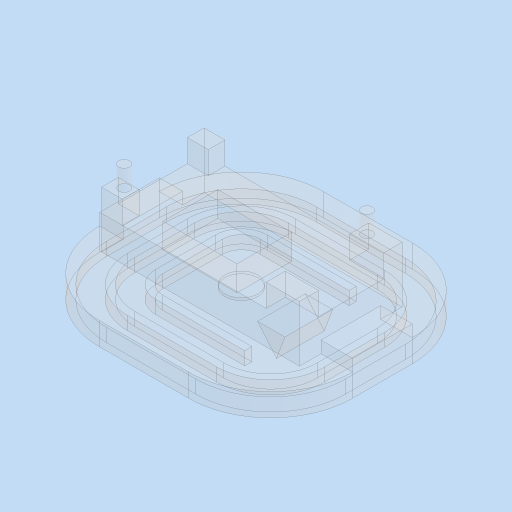
# Autodesk Inventor part: LM19-LSI_lens
Saved by Autodesk Inventor 2024 (Build 280153000, 153)
## iProperties
Created: 2025-05-08
Part Number: LM19-LSI_lens
Material: Polycarbonate, Clear
Document SubType Name: Modeling
Designer: XxPan
Density: 1.2 g/cm^3
Appearance: Polycarbonate - Clear
Author: XxPan
Autodesk Inventor part; units mm, degrees
ref_plane "YZ Plane" through (0, 0, 0) normal (1, 0, 0) x (0, 1, 0)
ref_plane "XZ Plane" through (0, 0, 0) normal (0, 1, 0) x (-1, 0, 0)
sketch "Sketch1" plane through (0, 0, 0) normal (0, 1, 0) x (-1, 0, 0)
  line L0 (3.725, 9.375) -> (-3.725, 9.375)
  line L1 (-10.6, 2.5) -> (-10.6, -2.5)
  line L2 (-3.725, -9.375) -> (3.725, -9.375)
  line L3 (10.6, -2.5) -> (10.6, 2.5)
  line L4 (16.8334, 0) -> (-16.8334, 0) construction
  line L5 (0, -15.1184) -> (0, 15.1184) construction
  arc A0 (10.6, 2.5) -> (3.725, 9.375) centre (3.725, 2.5) ccw
  arc A1 (3.725, -9.375) -> (10.6, -2.5) centre (3.725, -2.5) ccw
  arc A2 (-10.6, -2.5) -> (-3.725, -9.375) centre (-3.725, -2.5) ccw
  arc A3 (-3.725, 9.375) -> (-10.6, 2.5) centre (-3.725, 2.5) ccw
  point P0 (0, 0)
  point P1 (-10.6, -9.375)
  point P2 (-10.6, 9.375)
  point P3 (10.6, -9.375)
  dimension "d0" = 21.2
  dimension "d1" = 18.75
  dimension "d2" = 6.875
  constraints: 8 end point, 8 point on circle, 8 tangent, 6 point on line, 4 centre point, 3 equal radius, 2 parallel, 1 horizontal, 1 perpendicular, 2 other
  measures "d0" distance of point (10.6, -9.375) point (-10.6, -9.375)
  measures "d1" distance of point (-10.6, -9.375) point (-10.6, 9.375)
  measures "d2" radius of A0
extrude "Extrusion1" add sketch "Sketch1" against normal blind 0.8
sketch "Sketch2" plane through (0, -0.8, 0) normal (0, -1, 0) x (1, 0, 0)
  line L0 (10.6, -2.5) -> (10.6, 2.5) projected
  arc A0 (10.6, 2.5) -> (3.725, 9.375) centre (3.725, 2.5) ccw projected
  arc A1 (3.725, -9.375) -> (10.6, -2.5) centre (3.725, -2.5) ccw projected
  line L1 (-3.725, -9.375) -> (3.725, -9.375) projected
  arc A2 (-10.6, -2.5) -> (-3.725, -9.375) centre (-3.725, -2.5) ccw projected
  line L2 (-10.6, 2.5) -> (-10.6, -2.5) projected
  arc A3 (-3.725, 9.375) -> (-10.6, 2.5) centre (-3.725, 2.5) ccw projected
  line L3 (3.725, 9.375) -> (-3.725, 9.375) projected
  arc A4 (10, 2.5) -> (3.725, 8.775) centre (3.725, 2.5) ccw
  line L4 (10, 2.5) -> (10, -2.5)
  arc A5 (3.725, -8.775) -> (10, -2.5) centre (3.725, -2.5) ccw
  line L5 (3.725, -8.775) -> (-3.725, -8.775)
  arc A6 (-10, -2.5) -> (-3.725, -8.775) centre (-3.725, -2.5) ccw
  line L6 (-10, -2.5) -> (-10, 2.5)
  arc A7 (-3.725, 8.775) -> (-10, 2.5) centre (-3.725, 2.5) ccw
  line L7 (-3.725, 8.775) -> (3.725, 8.775)
  arc A8 (8.25, 2.5) -> (3.725, 7.025) centre (3.725, 2.5) ccw
  line L8 (8.25, 2.5) -> (8.25, -2.5)
  arc A9 (3.725, -7.025) -> (8.25, -2.5) centre (3.725, -2.5) ccw
  line L9 (3.725, -7.025) -> (-3.725, -7.025)
  arc A10 (-8.25, -2.5) -> (-3.725, -7.025) centre (-3.725, -2.5) ccw
  line L10 (-8.25, -2.5) -> (-8.25, 2.5)
  arc A11 (-3.725, 7.025) -> (-8.25, 2.5) centre (-3.725, 2.5) ccw
  line L11 (-3.725, 7.025) -> (3.725, 7.025)
  arc A12 (7.65, 2.5) -> (3.725, 6.425) centre (3.725, 2.5) ccw
  line L12 (7.65, 2.5) -> (7.65, -2.5)
  arc A13 (3.725, -6.425) -> (7.65, -2.5) centre (3.725, -2.5) ccw
  line L13 (3.725, -6.425) -> (-3.725, -6.425)
  arc A14 (-7.65, -2.5) -> (-3.725, -6.425) centre (-3.725, -2.5) ccw
  line L14 (-7.65, -2.5) -> (-7.65, 2.5)
  arc A15 (-3.725, 6.425) -> (-7.65, 2.5) centre (-3.725, 2.5) ccw
  line L15 (-3.725, 6.425) -> (3.725, 6.425)
  arc A16 (5.9, 2.5) -> (3.725, 4.675) centre (3.725, 2.5) ccw
  line L16 (5.9, 2.5) -> (5.9, -2.5)
  arc A17 (3.725, -4.675) -> (5.9, -2.5) centre (3.725, -2.5) ccw
  line L17 (3.725, -4.675) -> (-3.725, -4.675)
  arc A18 (-5.9, -2.5) -> (-3.725, -4.675) centre (-3.725, -2.5) ccw
  line L18 (-5.9, -2.5) -> (-5.9, 2.5)
  arc A19 (-3.725, 4.675) -> (-5.9, 2.5) centre (-3.725, 2.5) ccw
  line L19 (-3.725, 4.675) -> (3.725, 4.675)
  arc A20 (5.3, 2.5) -> (3.725, 4.075) centre (3.725, 2.5) ccw
  line L20 (5.3, 2.5) -> (5.3, -2.5)
  arc A21 (3.725, -4.075) -> (5.3, -2.5) centre (3.725, -2.5) ccw
  line L21 (3.725, -4.075) -> (-3.725, -4.075)
  arc A22 (-5.3, -2.5) -> (-3.725, -4.075) centre (-3.725, -2.5) ccw
  line L22 (-5.3, -2.5) -> (-5.3, 2.5)
  arc A23 (-3.725, 4.075) -> (-5.3, 2.5) centre (-3.725, 2.5) ccw
  line L23 (-3.725, 4.075) -> (3.725, 4.075)
  line L24 (3.725, 4.075) -> (3.725, 4.675)
  line L25 (3.725, -4.075) -> (3.725, -4.675)
  point P0 (0, 0)
  dimension "d5" = 0.6
  dimension "d6" = 1.75
  dimension "d7" = 0.6
  dimension "d8" = 1.75
  dimension "d9" = 0.6
  constraints: 44 end point, 40 point on circle, 20 centre point, 35 other
  measures "d5" radial gap between concentric circles of A0 A4
  measures "d6" radial gap between concentric circles of A4 A8
  measures "d7" radial gap between concentric circles of A8 A12
  measures "d8" radial gap between concentric circles of A12 A16
  measures "d9" radial gap between concentric circles of A16 A20
extrude "Extrusion2" add sketch "Sketch2" along normal blind 1.1 contours A1 L1 A2 L2 A3 L3 A0 L0 | L8 A9 L9 A10 L10 A11 L11 A8 | L24 L23 A23 L22 A22 L21 L25 L17 A18 L18 A19 L19
sketch "Sketch3" plane through (0, 0, 0) normal (0, 1, 0) x (1, 0, 0)
  line L0 (7.95, 4.3) -> (-8.65, 4.3)
  line L1 (-8.65, 4.3) -> (-8.65, -4.3)
  line L2 (-8.65, -4.3) -> (7.95, -4.3)
  line L3 (7.95, -4.3) -> (7.95, 4.3)
  line L4 (-14.84, 0) -> (14.84, 0) construction
  line L5 (-10.6, 2.5) -> (-10.6, -2.5) projected
  point P0 (0, 0)
  dimension "d12" = 16.6
  dimension "d13" = 8.6
  dimension "d14" = 1.95
  constraints: 8 end point, 2 parallel, 1 horizontal, 1 perpendicular, 1 other
  measures "d12" distance of L2.end L1.end
  measures "d13" distance of L1.end L0.end
  measures "d14" distance between parallel lines of L5 L1
extrude "Extrusion3" add sketch "Sketch3" along normal blind 2.8
sketch "Sketch4" plane through (0, 2.8, 0) normal (0, 1, 0) x (1, 0, 0)
  line L0 (0.7, 2.3) -> (-5.5, 2.3)
  line L1 (-5.5, 2.3) -> (-5.5, -2.3)
  line L2 (-5.5, -2.3) -> (0.7, -2.3)
  line L3 (0.7, -2.3) -> (0.7, 2.3)
  line L4 (-14.84, 0) -> (14.84, 0) construction
  line L5 (-8.65, 4.3) -> (-8.65, -4.3) projected
  point P0 (0, 0)
  dimension "d17" = 6.2
  dimension "d18" = 4.6
  dimension "d19" = 3.15
  constraints: 8 end point, 2 parallel, 1 horizontal, 1 perpendicular, 1 other
  measures "d17" distance of L2.end L1.end
  measures "d18" distance of L1.end L0.end
  measures "d19" distance between parallel lines of L5 L1
extrude "Extrusion4" cut sketch "Sketch4" against normal blind 2.1
sketch "Sketch5" plane through (0, 2.8, 0) normal (0, 1, 0) x (1, 0, 0)
  line L0 (-8.65, 4.3) -> (7.95, 4.3) projected
  line L1 (7.95, 4.3) -> (5.15, 4.3)
  line L2 (5.15, 4.3) -> (5.15, 2.7)
  line L3 (5.15, 2.7) -> (7.95, 2.7)
  line L4 (7.95, 2.7) -> (7.95, 4.3)
  line L5 (-8.65, -4.3) -> (7.95, -4.3) projected
  line L6 (7.95, -4.3) -> (5.15, -4.3)
  line L7 (5.15, -4.3) -> (5.15, -2.7)
  line L8 (5.15, -2.7) -> (7.95, -2.7)
  line L9 (7.95, -2.7) -> (7.95, -4.3)
  line L10 (-8.65, 4.3) -> (-8.65, -4.3) projected
  line L11 (-8.65, -4.3) -> (-6.9, -4.3)
  line L12 (-6.9, -4.3) -> (-6.9, -2.9)
  line L13 (-6.9, -2.9) -> (-8.65, -2.9)
  line L14 (-8.65, -2.9) -> (-8.65, -4.3)
  line L15 (-8.65, 4.3) -> (-6.9, 4.3)
  line L16 (-6.9, 4.3) -> (-6.9, 2.9)
  line L17 (-6.9, 2.9) -> (-8.65, 2.9)
  line L18 (-8.65, 2.9) -> (-8.65, 4.3)
  point P0 (0, 0)
  dimension "d22" = 2.8
  dimension "d23" = 1.6
  dimension "d24" = 2.8
  dimension "d25" = 1.6
  dimension "d26" = 1.75
  dimension "d27" = 1.4
  dimension "d28" = 1.75
  dimension "d29" = 1.4
  constraints: 32 end point, 8 parallel, 4 horizontal, 4 perpendicular
  measures "d22" distance of L3.end L2.end
  measures "d23" distance of L2.end L1.end
  measures "d24" distance of L7.end L8.end
  measures "d25" distance of L6.end L7.end
  measures "d26" distance of L13.end L12.end
  measures "d27" distance of L12.end L11.end
  measures "d28" distance of L16.end L17.end
  measures "d29" distance of L15.end L16.end
extrude "Extrusion5" add sketch "Sketch5" along normal blind 1.9
sketch "Sketch6" plane through (0, 0, 0) normal (0, 1, 0) x (1, 0, 0)
  arc A0 (-3.725, 9.375) -> (-10.6, 2.5) centre (-3.725, 2.5) ccw projected
  line L0 (-8.65, -4.3) -> (-8.65, 4.3) projected
  line L1 (-10.6, 2.5) -> (-8.65, 2.5)
  line L2 (-8.65, 2.5) -> (-8.65, -2.5)
  line L3 (-8.65, -2.5) -> (-10.6, -2.5)
  line L4 (-10.6, -2.5) -> (-10.6, 2.5)
  line L5 (10.6, 2.5) -> (10.6, -2.5) projected
  line L6 (7.95, 4.3) -> (7.95, -4.3) projected
  line L7 (10.6, 2.5) -> (7.95, 2.5)
  line L8 (7.95, 2.5) -> (7.95, -2.5)
  line L9 (7.95, -2.5) -> (10.6, -2.5)
  line L10 (10.6, -2.5) -> (10.6, 2.5)
  point P0 (0, 0)
  dimension "d32" = 5
  dimension "d33" = 5
  constraints: 16 end point, 4 parallel, 2 horizontal, 2 perpendicular, 2 point on line
  measures "d32" distance of L1.end L2.end
  measures "d33" distance of L8.end L7.end
extrude "Extrusion6" add sketch "Sketch6" along normal blind 1
sketch "Sketch7" plane through (0, 4.7, 0) normal (0, 1, 0) x (1, 0, 0)
  circle A0 centre (5.9, 3.415) radius 0.45
  circle A1 centre (-7.64, -3.415) radius 0.45
  line L0 (5.15, 4.3) -> (5.15, 2.7) projected
  line L1 (-6.9, -4.3) -> (-6.9, -2.9) projected
  line L2 (5.15, 2.7) -> (7.95, 2.7) projected
  line L3 (-6.9, -2.9) -> (-8.65, -2.9) projected
  point P0 (0, 0)
  point P1 (5.15, 3.5)
  point P2 (-6.9, -3.6)
  point P3 (6.55, 2.7)
  point P4 (-7.775, -2.9)
  dimension "d36" = 0.9
  dimension "d37" = 0.9
  dimension "d48" = 13.54
  dimension "d49" = 6.83
  dimension "d50" = 3.415
  dimension "d52" = 5.9
  constraints: 4 midpoint, 2 centre point
  measures "d36" diameter of A0
  measures "d37" diameter of A1
  measures "d48" horizontal distance of A0.centre A1.centre
  measures "d49" vertical distance of A0.centre A1.centre
  measures "d50" vertical distance of point (0, 0) A1.centre
  measures "d52" horizontal distance of point (0, 0) A0.centre
extrude "Extrusion7" add sketch "Sketch7" along normal blind 1.75
ref_plane "Work Plane1" through (3.725, -0.8, 0) normal (0, 0, -1) x (-1, 0, 0)
sketch "Sketch8" plane through (3.725, -0.8, 0) normal (0, 0, -1) x (-1, 0, 0)
  line L0 (0, 0) -> (0, -1.1) construction
  line L1 (1.5943, 0) -> (0, -1.9)
  line L2 (0, -1.9) -> (-0.6915, 0)
  line L3 (7.45, -1.1) -> (0, -1.1) construction
  line L4 (0, 0) -> (7.45, 0) projected
  line L5 (-3.925, 0) -> (0, 0) projected
  point P0 (3.725, 0.8)
  dimension "d40" = 0.8
  dimension "d41" = 60
  dimension "d42" = 70
  constraints: 4 end point, 3 point on line
  measures "d40" distance from line of L3 L1.end
  measures "d41" angle of L2 L1
  measures "d42" angle of L5 L2
extrude "Extrusion8" add sketch "Sketch8" along normal mid plane 4
sketch "Sketch9" plane through (0, -0.8, 0) normal (0, -1, 0) x (1, 0, 0)
  circle A0 centre (-1.225, 0) radius 1.375
  arc A1 (-3.725, 4.075) -> (-5.3, 2.5) centre (-3.725, 2.5) ccw projected
  arc A2 (-5.3, -2.5) -> (-3.725, -4.075) centre (-3.725, -2.5) ccw projected
  line L0 (-3.725, 2.5) -> (-1.225, 0) construction
  line L1 (-1.225, 0) -> (-3.725, -2.5) construction
  point P0 (0, 0)
  dimension "d45" = 2.75
  constraints: 4 end point, 1 centre point, 1 coincident, 1 horizontal alignment, 1 perpendicular
  measures "d45" diameter of A0
extrude "Extrusion9" add sketch "Sketch9" along normal blind 0.2
equation "\"d29\" = d27"
equation "\"d50\" = 0.5 * d49"
body "Solid1"
